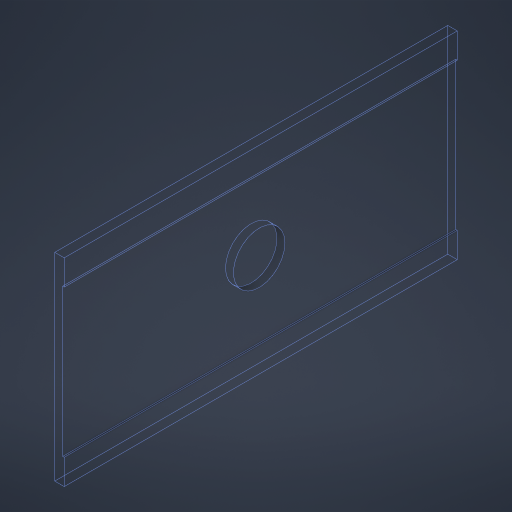
# Autodesk Inventor part: Osnova
Saved by Autodesk Inventor 2024 (Build 280153000, 153)
## iProperties
Created: 2023-12-23
Part Number: Osnova
Material: Aluminum 6061
Document SubType Name: Modeling
Designer: KirikDK
Mass: 3429.82 g
Surface Area: 2625.49 cm^2
Volume: 1270.3 cm^3
Density: 2.7 g/cm^3
Appearance: Aluminum - Flat
Author: KirikDK
Autodesk Inventor part; units mm, degrees
ref_plane "YZ Plane" through (0, 0, 0) normal (1, 0, 0) x (0, 1, 0)
ref_plane "XZ Plane" through (0, 0, 0) normal (0, 1, 0) x (-1, 0, 0)
ref_plane "XY Plane" through (0, 0, 0) normal (0, 0, 1) x (1, 0, 0)
sketch "Sketch1" plane through (0, 0, 0) normal (0, 1, 0) x (-1, 0, 0)
  line L0 (95, 271.4286) -> (85, 271.4286)
  line L1 (85, 271.4286) -> (85, -224.5714)
  line L2 (85, -224.5714) -> (95, -224.5714)
  line L3 (95, -224.5714) -> (95, 271.4286)
  point P0 (0, 0)
  dimension "d0" = 10
  dimension "d1" = 496
  constraints: 8 end point, 2 parallel, 1 horizontal, 1 perpendicular
  measures "d0" distance of L0.start L0.end
  measures "d1" distance of L2.end L0.start
extrude "Extrusion1" add sketch "Sketch1" along normal blind 250
sketch "Sketch2" plane through (-85, 0, 271.4286) normal (1, 0, 0) x (0, 0, -1)
  line L0 (0, 0) -> (0, 250) projected
  line L1 (496, 0) -> (496, 250) projected
  line L2 (0, 218) -> (496, 218)
  line L3 (496, 218) -> (496, 32)
  line L4 (496, 32) -> (0, 32)
  line L5 (0, 32) -> (0, 218)
  line L6 (0, 250) -> (496, 250) projected
  line L7 (0, 0) -> (496, 0) projected
  point P0 (271.4286, 0)
  point P1 (0, 32)
  point P2 (496, 218)
  dimension "d4" = 32
  dimension "d5" = 32
  dimension "d6" = 186
  constraints: 8 end point, 2 parallel, 2 point on line, 1 horizontal, 1 perpendicular
  measures "d4" distance between parallel lines of L6 L2
  measures "d5" distance between parallel lines of L7 L4
  measures "d6" distance between parallel lines of L2 L4
extrude "Extrusion3" add sketch "Sketch2" along normal blind 2 contours L0 L4 L1 L7 | L0 L6 L1 L2
sketch "Sketch3" plane through (-95, 0, -224.5714) normal (-1, 0, 0) x (0, 0, 1)
  line L0 (0, 250) -> (496, 250) projected
  circle A0 centre (248, 250) radius 8
  line L1 (496, 32) -> (496, 218) projected
  circle A1 centre (496, 125) radius 12
  circle A2 centre (248, 125) radius 32.5
  point P0 (224.5714, 0)
  dimension "d11" = 65
  constraints: 3 centre point, 2 midpoint
  measures "d11" diameter of A2
extrude "Extrusion4" cut sketch "Sketch3" against normal blind 35 contours A2
body "Solid1"
